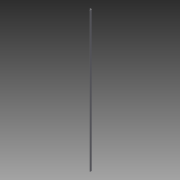
# Autodesk Inventor part: Angle Iron-01
Saved by Autodesk Inventor 2013 (Build 170138000, 138)
## iProperties
Created: 2012-10-17
Part Number: Angle Iron-01
Material: Generic
Document SubType Name: Modeling
Designer: Istvan
Density: 1 g/cm^3
Author: Istvan
Autodesk Inventor part; units mm, degrees
ref_plane "YZ Plane" through (0, 0, 0) normal (1, 0, 0) x (0, 1, 0)
ref_plane "XZ Plane" through (0, 0, 0) normal (0, 1, 0) x (-1, 0, 0)
ref_plane "XY Plane" through (0, 0, 0) normal (0, 0, 1) x (1, 0, 0)
sketch "Sketch1" plane through (0, 0, 0) normal (0, 1, 0) x (-1, 0, 0)
  line L0 (2.54, 0) -> (25.4, 0)
  line L1 (0, 25.4) -> (0, 2.54)
  line L2 (22.86, 4.7625) -> (7.3025, 4.7625)
  line L3 (4.7625, 7.3025) -> (4.7625, 22.86)
  line L4 (2.2225, 25.4) -> (0, 25.4)
  line L5 (25.4, 2.2225) -> (25.4, 0)
  arc A0 (4.7625, 7.3025) -> (7.3025, 4.7625) centre (7.3025, 7.3025) ccw
  arc A1 (4.7625, 22.86) -> (2.2225, 25.4) centre (2.2225, 22.86) ccw
  arc A2 (0, 2.54) -> (2.54, 0) centre (2.54, 2.54) ccw
  arc A3 (25.4, 2.2225) -> (22.86, 4.7625) centre (22.86, 2.2225) ccw
  point P0 (0, 0)
  dimension "d2" = 4.7625
  dimension "d3" = 25.4
  dimension "d4" = 25.4
  dimension "d5" = 2.54
  constraints: 12 end point, 8 point on circle, 8 tangent, 4 centre point, 3 equal radius, 3 perpendicular, 2 point on line, 1 horizontal, 1 other
  measures "d2" distance between parallel lines of L3 L1
  measures "d3" distance of point (0, 0) L0.end
  measures "d4" distance of L1.start point (0, 0)
  measures "d5" radius of A0
extrude "Angle Iron Template" add sketch "Sketch1" along normal blind 1828.8
body "Solid1"
